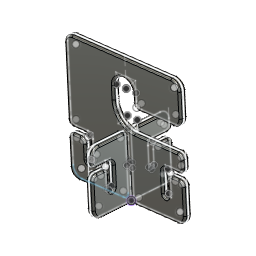
Earring Hanger (Autodesk Fusion 360 design; units mm, degrees)
Autodesk Fusion 360 part; units mm, degrees
sketch "Main shape" plane through (0, 0, 0) normal (0, 0, 1) x (1, 0, 0)
  line L0 (15, 35) -> (-15, 35) construction
  line L1 (-17.5, 32.5) -> (-17.5, 2.5) construction
  line L2 (-15, 0) -> (15, 0) construction
  line L3 (17.5, 2.5) -> (17.5, 32.5) construction
  line L4 (0, 35) -> (0, 0) construction
  line L5 (0, 20.5) -> (0, 27) construction
  line L6 (3, 30) -> (-3, 30) construction
  line L7 (-3, 30) -> (-3, 24) construction
  line L8 (-3, 24) -> (3, 24) construction
  line L9 (3, 24) -> (3, 30) construction
  line L10 (3, 30) -> (-3, 24) construction
  line L11 (-3, 30) -> (3, 24) construction
  line L12 (3, 23.5) -> (-3, 23.5) construction
  line L13 (-3, 23.5) -> (-3, 17.5) construction
  line L14 (-3, 17.5) -> (3, 17.5) construction
  line L15 (3, 17.5) -> (3, 23.5) construction
  line L16 (3, 23.5) -> (-3, 17.5) construction
  line L17 (-3, 23.5) -> (3, 17.5) construction
  line L18 (-11, 5) -> (-12.5, 5) construction
  line L19 (-12.5, 5) -> (-12.5, 6.5) construction
  line L20 (-12.5, 6.5) -> (-11, 6.5) construction
  line L21 (-11, 6.5) -> (-11, 5) construction
  line L22 (-11, 5) -> (-12.5, 6.5) construction
  line L23 (-12.5, 5) -> (-11, 6.5) construction
  line L24 (-11, 11) -> (-12.5, 11) construction
  line L25 (-12.5, 11) -> (-12.5, 12.5) construction
  line L26 (-12.5, 12.5) -> (-11, 12.5) construction
  line L27 (-11, 12.5) -> (-11, 11) construction
  line L28 (-11, 11) -> (-12.5, 12.5) construction
  line L29 (-12.5, 11) -> (-11, 12.5) construction
  line L30 (12.5, 11) -> (11, 11) construction
  line L31 (11, 11) -> (11, 12.5) construction
  line L32 (11, 12.5) -> (12.5, 12.5) construction
  line L33 (12.5, 12.5) -> (12.5, 11) construction
  line L34 (12.5, 11) -> (11, 12.5) construction
  line L35 (11, 11) -> (12.5, 12.5) construction
  line L36 (12.5, 5) -> (11, 5) construction
  line L37 (11, 5) -> (11, 6.5) construction
  line L38 (11, 6.5) -> (12.5, 6.5) construction
  line L39 (12.5, 6.5) -> (12.5, 5) construction
  line L40 (12.5, 5) -> (11, 6.5) construction
  line L41 (11, 5) -> (12.5, 6.5) construction
  arc A0 (-15, 35) -> (-17.5, 32.5) centre (-15, 32.5) ccw construction
  arc A1 (17.5, 32.5) -> (15, 35) centre (15, 32.5) ccw construction
  arc A2 (15, 0) -> (17.5, 2.5) centre (15, 2.5) ccw construction
  arc A3 (-17.5, 2.5) -> (-15, 0) centre (-15, 2.5) ccw construction
  line L42 (3, 27) -> (3, 25)
  line L43 (4.5, 23.5) -> (15, 23.5)
  line L44 (17.5, 26) -> (17.5, 32.5)
  line L45 (15, 35) -> (-15, 35)
  line L46 (12.5, 12.5) -> (16, 12.5)
  line L47 (11, 11) -> (11, 5.75)
  line L48 (12.5, 9.5) -> (12.5, 5.75)
  line L49 (14, 11) -> (16, 11)
  line L50 (-14, 11) -> (-16, 11)
  line L51 (-12.5, 9.5) -> (-12.5, 5.75)
  line L52 (-11, 11) -> (-11, 5.75)
  line L53 (17.5, 9.5) -> (17.5, 2.5)
  line L54 (-17.5, 14) -> (-17.5, 32.5)
  line L55 (-3, 27) -> (-3, 23.5)
  arc A4 (-11, 11) -> (-12.5, 12.5) centre (-12.5, 11) ccw
  arc A5 (12.5, 12.5) -> (11, 11) centre (12.5, 11) ccw
  arc A6 (11, 5.75) -> (12.5, 5.75) centre (11.75, 5.75) ccw
  arc A7 (-12.5, 5.75) -> (-11, 5.75) centre (-11.75, 5.75) ccw
  arc A8 (15, 0) -> (17.5, 2.5) centre (15, 2.5) ccw
  arc A9 (17.5, 32.5) -> (15, 35) centre (15, 32.5) ccw
  arc A10 (-15, 35) -> (-17.5, 32.5) centre (-15, 32.5) ccw
  arc A11 (3, 27) -> (-3, 27) centre (0, 27) ccw
  arc A12 (-3, 23.5) -> (3, 17.5) centre (3, 23.5) ccw
  line L56 (-16, 12.5) -> (-12.5, 12.5)
  arc A13 (15, 23.5) -> (17.5, 26) centre (15, 26) ccw
  line L57 (-17.5, 9.5) -> (-17.5, 2.5)
  arc A14 (-17.5, 2.5) -> (-15, 0) centre (-15, 2.5) ccw
  line L58 (3, 17.5) -> (16, 17.5)
  line L59 (17.5, 16) -> (17.5, 14)
  arc A15 (17.5, 16) -> (16, 17.5) centre (16, 16) ccw
  arc A16 (16, 12.5) -> (17.5, 14) centre (16, 14) ccw
  arc A17 (14, 11) -> (12.5, 9.5) centre (14, 9.5) ccw
  arc A18 (17.5, 9.5) -> (16, 11) centre (16, 9.5) ccw
  arc A19 (-12.5, 9.5) -> (-14, 11) centre (-14, 9.5) ccw
  arc A20 (-16, 11) -> (-17.5, 9.5) centre (-16, 9.5) ccw
  arc A21 (-17.5, 14) -> (-16, 12.5) centre (-16, 14) ccw
  arc A22 (3, 25) -> (4.5, 23.5) centre (4.5, 25) ccw
  line L60 (0, 0) -> (0, 9) construction
  line L61 (-0.85, 9) -> (0.85, 9) construction
  line L62 (0.85, 9) -> (0.85, 7.3) construction
  line L63 (0.85, 7.3) -> (-0.85, 7.3) construction
  line L64 (-0.85, 7.3) -> (-0.85, 9) construction
  arc A23 (0.85, 8.15) -> (-0.85, 8.15) centre (0, 8.15) ccw
  line L65 (-0.85, 8.15) -> (-0.85, 1.5)
  line L66 (0.85, 8.15) -> (0.85, 1.5)
  line L67 (-15, 0) -> (-2.35, 0)
  line L68 (2.35, 0) -> (15, 0)
  arc A24 (0.85, 1.5) -> (2.35, 0) centre (2.35, 1.5) ccw
  arc A25 (-2.35, 0) -> (-0.85, 1.5) centre (-2.35, 1.5) ccw
  point P0 (0, 27)
  point P1 (0, 20.5)
  point P2 (3, 27)
  point P3 (-3, 27)
  point P4 (-3, 20.5)
  point P5 (3, 20.5)
  point P6 (-11.75, 5.75)
  point P7 (-11.75, 11.75)
  point P8 (11.75, 11.75)
  point P9 (11.75, 5.75)
  point P10 (0, 9)
  point P11 (-0.85, 8.15)
  point P12 (0.85, 8.15)
  dimension "d21" = 35
  dimension "d22" = 35
  dimension "d25" = 6
  dimension "d28" = 5
  dimension "d29" = 17.5
  dimension "d30" = 1.5
  dimension "d31" = 5
  dimension "d32" = 12.5
  dimension "d33" = 5.75
  dimension "d35" = 2.5
  dimension "d38" = 2.5
  dimension "d41" = 1.5
  dimension "d97" = 9
  dimension "d98" = 1.7
  constraint horizontal L0
  constraint perpendicular L0 L1
  constraint parallel L0 L2
  constraint parallel L1 L3
  constraint coincident L4.end L60.start
  constraint coincident L4 P1
  constraint coincident L4 P0
  constraint horizontal L6
  constraint perpendicular L6 L7
  constraint parallel L6 L8
  constraint parallel L7 L9
  constraint coincident L10 P0
  constraint coincident L11 P0
  constraint coincident P0 L5.end
  constraint perpendicular L10 L11
  constraint horizontal L12
  constraint perpendicular L12 L13
  constraint parallel L12 L14
  constraint parallel L13 L15
  constraint coincident L16 P1
  constraint coincident L17 P1
  constraint coincident P1 L5.start
  constraint equal L7 L13
  constraint collinear L7 L13
  constraint midpoint L9 P2
  constraint midpoint L7 P3
  constraint midpoint L13 P4
  constraint midpoint L15 P5
  constraint horizontal L18
  constraint perpendicular L18 L19
  constraint parallel L18 L20
  constraint parallel L19 L21
  constraint coincident L22 P6
  constraint coincident L23 P6
  constraint perpendicular L22 L23
  constraint horizontal L24
  constraint perpendicular L24 L25
  constraint parallel L24 L26
  constraint parallel L25 L27
  constraint coincident L28 P7
  constraint coincident L29 P7
  constraint perpendicular L28 L29
  constraint collinear L21 L27
  constraint collinear L19 L25
  constraint horizontal L30
  constraint perpendicular L30 L31
  constraint parallel L30 L32
  constraint parallel L31 L33
  constraint coincident L34 P8
  constraint coincident L35 P8
  constraint perpendicular L34 L35
  constraint collinear L26 L32
  constraint horizontal L36
  constraint perpendicular L36 L37
  constraint parallel L36 L38
  constraint parallel L37 L39
  constraint coincident L40 P9
  constraint coincident L41 P9
  constraint perpendicular L40 L41
  constraint collinear L24 L30
  constraint collinear L20 L38
  constraint collinear L18 L36
  constraint collinear L33 L39
  constraint symmetric L4 P7 P8
  constraint coincident L0 L4.start
  constraint tangent L0 A0
  constraint tangent L1 A0
  constraint tangent L3 A1
  constraint tangent L0 A1
  constraint coincident L2 L4.end
  constraint tangent L3 A2
  constraint tangent L2 A2
  constraint tangent L1 A3
  constraint tangent L2 A3
  constraint equal A0 A1
  constraint equal A0 A3
  constraint equal A2 A3
  constraint coincident P2 L42.start
  constraint perpendicular L3 L43
  constraint perpendicular L3 L46
  constraint midpoint L37 L47.end
  constraint midpoint L39 L48.end
  constraint perpendicular L3 L49
  constraint perpendicular L1 L50
  constraint midpoint L19 L51.end
  constraint midpoint L21 L52.end
  constraint coincident P3 L55.start
  constraint tangent L26 A4
  constraint tangent L32 A5
  constraint tangent L36 A6
  constraint tangent L18 A7
  constraint tangent L3 A8
  constraint tangent L3 A9
  constraint tangent L54 A10
  constraint tangent L6 A11
  constraint tangent L14 A12
  constraint tangent A4 L56
  constraint tangent L43 A13
  constraint tangent L44 A13
  constraint collinear L3 L44
  constraint tangent L58 A15
  constraint tangent L59 A15
  constraint tangent L46 A16
  constraint tangent L59 A16
  constraint coincident L30.start L49
  constraint coincident L30.start L48
  constraint tangent L49 A17
  constraint tangent L48 A17
  constraint equal A16 A17
  constraint tangent L53 A18
  constraint tangent L49 A18
  constraint equal A16 A18
  constraint collinear L3 L53
  constraint coincident L24.end L51
  constraint tangent L50 A19
  constraint tangent L51 A19
  constraint equal A17 A19
  constraint tangent L50 A20
  constraint tangent L57 A20
  constraint equal A19 A20
  constraint tangent L54 A21
  constraint tangent L56 A21
  constraint equal A20 A21
  constraint equal A15 A16
  constraint collinear L49 L50
  constraint collinear L3 L59
  constraint horizontal L58
  constraint collinear L1 L54
  constraint coincident L12.start L42
  constraint coincident L12.start L43
  constraint tangent L42 A22
  constraint tangent L43 A22
  constraint equal A15 A22
  constraint collinear L1 L57
  constraint coincident L4 P10
  constraint horizontal L61
  constraint vertical L62
  constraint horizontal L63
  constraint vertical L64
  constraint equal L61 L64
  constraint midpoint L61 P10
  constraint midpoint L64 P11
  constraint midpoint L62 P12
  constraint coincident P10 L60.end
  constraint coincident P11 A23.end
  constraint coincident P10 A23
  constraint tangent L61 A23
  constraint coincident P12 A23.start
  constraint tangent A23 L65
  constraint perpendicular L2 L65
  constraint tangent A23 L66
  constraint tangent L66 A24
  constraint tangent L68 A24
  constraint equal A16 A24
  constraint collinear L2 L68
  constraint tangent L65 A25
  constraint tangent L67 A25
  constraint equal A24 A25
  measures "d21" distance of L0 L2
  measures "d22" distance of L1 L3
  measures "d25" distance of L7 L9
  measures "d28" distance of L0 L6
  measures "d29" distance of L0 L14
  measures "d30" distance of L19 L21
  measures "d31" distance of L2 L18
  measures "d32" distance of L2 L26
  measures "d33" distance of L1 P6
  measures "d35" radius of A1
  measures "d38" radius of A13
  measures "d41" radius of A16
  measures "d97" distance of L4.end P10
  measures "d98" distance of L62 L64
sketch "Adapter shape" plane through (0, 0, 0) normal (1, 0, 0) x (0, 1, 0)
  line L0 (0, 0) -> (17.5, 0)
  line L1 (0, 12.125) -> (17.5, 12.125) construction
  line L2 (17.5, 12.125) -> (17.5, -9.625) construction
  line L3 (17.5, -12.125) -> (0, -12.125) construction
  line L4 (0, -12.125) -> (0, 12.125) construction
  line L5 (11, 7.125) -> (12.5, 7.125) construction
  line L6 (12.5, 7.125) -> (12.5, 5.625) construction
  line L7 (12.5, 5.625) -> (11, 5.625) construction
  line L8 (11, 5.625) -> (11, 7.125) construction
  line L9 (5, 7.125) -> (6.5, 7.125) construction
  line L10 (6.5, 7.125) -> (6.5, 5.625) construction
  line L11 (6.5, 5.625) -> (5, 5.625) construction
  line L12 (5, 5.625) -> (5, 7.125) construction
  line L13 (5, -5.625) -> (6.5, -5.625) construction
  line L14 (6.5, -5.625) -> (6.5, -7.125) construction
  line L15 (6.5, -7.125) -> (5, -7.125) construction
  line L16 (5, -7.125) -> (5, -5.625) construction
  line L17 (11, -5.625) -> (12.5, -5.625) construction
  line L18 (12.5, -5.625) -> (12.5, -7.125) construction
  line L19 (12.5, -7.125) -> (11, -7.125) construction
  line L20 (11, -7.125) -> (11, -5.625) construction
  line L21 (11.75, 7.125) -> (11.75, 12.125) construction
  line L22 (11.75, -12.125) -> (11.75, -7.125) construction
  line L23 (9.7, 0.85) -> (8, 0.85) construction
  line L24 (8, 0.85) -> (8, -0.85) construction
  line L25 (8, -0.85) -> (9.7, -0.85) construction
  line L26 (9.7, -0.85) -> (9.7, 0.85) construction
  line L27 (9.7, 0.85) -> (8, -0.85) construction
  line L28 (11, 8.625) -> (11, 10.625)
  line L29 (9.5, 12.125) -> (2.5, 12.125)
  line L30 (9.5, 7.125) -> (5.75, 7.125)
  line L31 (14, 12.125) -> (15, 12.125)
  line L32 (9.7, 0) -> (8, 0) construction
  line L33 (8.85, 0.85) -> (16, 0.85)
  line L34 (17.5, 2.35) -> (17.5, 9.625)
  line L35 (8.85, -0.85) -> (16, -0.85)
  line L36 (5.75, -7.125) -> (9.5, -7.125)
  line L37 (11, -8.625) -> (11, -10.625)
  line L38 (9.5, -12.125) -> (2.5, -12.125)
  line L39 (0, 9.625) -> (0, -9.625)
  arc A0 (5.75, 7.125) -> (5.75, 5.625) centre (5.75, 6.375) ccw
  arc A1 (5.75, -5.625) -> (5.75, -7.125) centre (5.75, -6.375) ccw
  line L40 (14, -12.125) -> (15, -12.125)
  line L41 (12.5, 10.625) -> (12.5, 7.125)
  line L42 (5.75, 5.625) -> (11, 5.625)
  line L43 (5.75, -5.625) -> (11, -5.625)
  line L44 (12.5, -10.625) -> (12.5, -7.125)
  arc A2 (11, 5.625) -> (12.5, 7.125) centre (11, 7.125) ccw
  arc A3 (12.5, -7.125) -> (11, -5.625) centre (11, -7.125) ccw
  arc A4 (8.85, 0.85) -> (8.85, -0.85) centre (8.85, 0) ccw
  arc A5 (15, -12.125) -> (17.5, -9.625) centre (15, -9.625) ccw
  line L45 (17.5, -9.625) -> (17.5, -2.35)
  arc A6 (17.5, 9.625) -> (15, 12.125) centre (15, 9.625) ccw
  arc A7 (2.5, 12.125) -> (0, 9.625) centre (2.5, 9.625) ccw
  arc A8 (0, -9.625) -> (2.5, -12.125) centre (2.5, -9.625) ccw
  arc A9 (17.5, -2.35) -> (16, -0.85) centre (16, -2.35) ccw
  arc A10 (16, 0.85) -> (17.5, 2.35) centre (16, 2.35) ccw
  arc A11 (14, 12.125) -> (12.5, 10.625) centre (14, 10.625) ccw
  arc A12 (11, 10.625) -> (9.5, 12.125) centre (9.5, 10.625) ccw
  arc A13 (9.5, 7.125) -> (11, 8.625) centre (9.5, 8.625) ccw
  arc A14 (11, -8.625) -> (9.5, -7.125) centre (9.5, -8.625) ccw
  arc A15 (9.5, -12.125) -> (11, -10.625) centre (9.5, -10.625) ccw
  arc A16 (12.5, -10.625) -> (14, -12.125) centre (14, -10.625) ccw
  point P0 (17.5, 0)
  point P1 (11.75, -7.125)
  point P2 (8.85, 0)
  point P3 (9.7, 0)
  point P4 (5.75, 7.125)
  point P5 (5.75, 5.625)
  point P6 (5, 6.375)
  point P7 (5.75, -5.625)
  point P8 (5.75, -7.125)
  point P9 (5, -6.375)
  point P10 (8.85, 0.85)
  point P11 (8.85, -0.85)
  point P12 (8, 0)
  dimension "d61" = 17.5
  dimension "d62" = 24.25
  dimension "d63" = 1.5
  dimension "d64" = 12.5
  dimension "d65" = 5
  dimension "d66" = 5
  dimension "d68" = 1.7
  dimension "d71" = 2.5
  dimension "d75" = 1.5
  dimension "d103" = 9.5
  constraint coincident L0.start origin
  constraint horizontal L0
  constraint horizontal L1
  constraint vertical L2
  constraint horizontal L3
  constraint vertical L4
  constraint midpoint L4 L0.start
  constraint coincident P0 L0.end
  constraint horizontal L5
  constraint vertical L6
  constraint horizontal L7
  constraint vertical L8
  constraint equal L5 L8
  constraint horizontal L9
  constraint vertical L10
  constraint horizontal L11
  constraint vertical L12
  constraint equal L9 L12
  constraint collinear L5 L9
  constraint collinear L7 L11
  constraint horizontal L13
  constraint vertical L14
  constraint horizontal L15
  constraint vertical L16
  constraint equal L11 L13
  constraint equal L10 L14
  constraint horizontal L17
  constraint vertical L18
  constraint horizontal L19
  constraint vertical L20
  constraint equal L5 L17
  constraint equal L6 L18
  constraint collinear L12 L16
  constraint collinear L8 L20
  constraint midpoint L5 L21.start
  constraint coincident L1 L21.end
  constraint perpendicular L1 L21
  constraint coincident L3 L22.start
  constraint perpendicular L3 L22
  constraint equal L21 L22
  constraint collinear L21 L22
  constraint midpoint L19 P1
  constraint coincident P1 L22.end
  constraint collinear L15 L19
  constraint horizontal L23
  constraint vertical L24
  constraint horizontal L25
  constraint vertical L26
  constraint equal L23 L26
  constraint midpoint L27 P2
  constraint midpoint L26 P3
  constraint perpendicular L1 L28
  constraint midpoint L9 P4
  constraint midpoint L11 P5
  constraint midpoint L12 P6
  constraint midpoint L13 P7
  constraint midpoint L15 P8
  constraint midpoint L16 P9
  constraint coincident P4 L30.end
  constraint coincident P5 A0.end
  constraint midpoint L23 P10
  constraint midpoint L25 P11
  constraint midpoint L24 P12
  constraint coincident P3 L32.start
  constraint coincident P12 L32.end
  constraint collinear L0 L32
  constraint coincident P10 L33.start
  constraint perpendicular L2 L33
  constraint coincident P11 L35.start
  constraint perpendicular L2 L35
  constraint coincident P8 L36.start
  constraint perpendicular L3 L37
  constraint coincident P6 A0
  constraint tangent L12 A0
  constraint coincident P9 A1
  constraint tangent L16 A1
  constraint coincident P7 A1.start
  constraint perpendicular L5 L41
  constraint perpendicular L19 L44
  constraint tangent L7 A2
  constraint tangent L17 A3
  constraint coincident P12 A4
  constraint tangent L24 A4
  constraint coincident L2 P0
  constraint coincident L3.start L2
  constraint tangent L2 A5
  constraint tangent L40 A5
  constraint coincident L1.end L31
  constraint coincident L1.end L34
  constraint tangent L31 A6
  constraint tangent L34 A6
  constraint coincident L1.start L29
  constraint coincident L1.start L39
  constraint tangent L29 A7
  constraint tangent L39 A7
  constraint coincident L3.end L39
  constraint coincident L3.end L38
  constraint tangent L39 A8
  constraint tangent L38 A8
  constraint equal A5 A6
  constraint equal A6 A7
  constraint equal A7 A8
  constraint tangent L45 A9
  constraint tangent L35 A9
  constraint tangent L33 A10
  constraint tangent L34 A10
  constraint tangent L31 A11
  constraint tangent L41 A11
  constraint tangent L28 A12
  constraint tangent L29 A12
  constraint coincident L5.start L28
  constraint coincident L5.start L30
  constraint tangent L28 A13
  constraint tangent L30 A13
  constraint coincident L19.end L36
  constraint coincident L19.end L37
  constraint tangent L36 A14
  constraint tangent L37 A14
  constraint tangent L37 A15
  constraint tangent L38 A15
  constraint tangent L44 A16
  constraint tangent L40 A16
  constraint equal A9 A10
  constraint equal A10 A11
  constraint equal A11 A12
  constraint equal A12 A13
  constraint equal A13 A15
  constraint equal A14 A15
  constraint equal A14 A16
  constraint collinear L3 L40
  constraint collinear L3 L38
  constraint collinear L2 L34
  constraint collinear L1 L31
  constraint collinear L1 L29
  constraint vertical L45
  measures "d61" distance of P0 L0.start
  measures "d62" distance of L1 L3
  measures "d63" distance of L5 L7
  measures "d64" distance of L4 L6
  measures "d65" distance of L4 L12
  measures "d66" distance of L1 L5
  measures "d68" distance of L23 L25
  measures "d71" radius of A5
  measures "d75" radius of A9
  measures "d103" distance of L2 L24
extrude "Extrude5" add sketch "Main shape" along normal mid plane 2 makes body 1
extrude "Extrude6" add sketch "Adapter shape" along normal mid plane 2 separate body makes body 2
fillet "Fillet4" radius 0.5 4 faces at (-12.6667, 23.3333, 1) (-12.6667, 23.3333, -1) (1, 1.7212, 1.9691) (-1, 1.7212, 1.9691) on bodies 1 2
named bodies: "Main", "Adapter"
